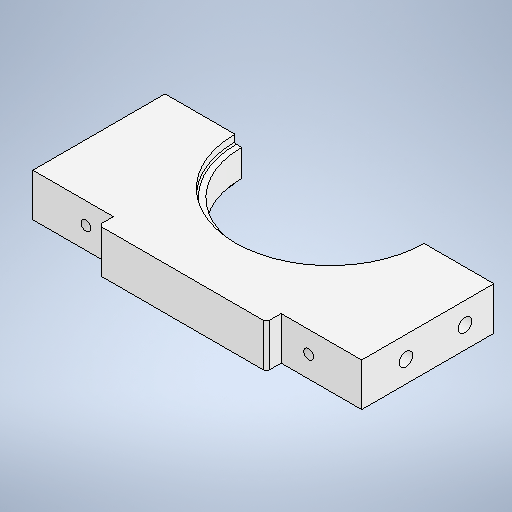
# Autodesk Inventor part: joint3_frame2
Saved by Autodesk Inventor 2025.3 (Build 293356030, 356C)
## iProperties
Created: 2025-11-25
Part Number: joint3_frame2
Material: PLA filament
Document SubType Name: Modeling
Designer: MSI
Density: 1.2 g/cm^3
Appearance: 일반
Mass: 86.6574 g
Surface Area: 168.952 cm^2
Volume: 72.2145 cm^3
Author: MSI
Autodesk Inventor part; units mm, degrees
ref_plane "YZ Plane" through (0, 0, 0) normal (1, 0, 0) x (0, 1, 0)
ref_plane "XZ Plane" through (0, 0, 0) normal (0, 1, 0) x (-1, 0, 0)
ref_plane "XY Plane" through (0, 0, 0) normal (0, 0, 1) x (1, 0, 0)
sketch "스케치1" plane through (0, 0, 0) normal (0, 1, 0) x (-1, 0, 0)
  line L0 (123, 55) -> (-123, 55)
  line L1 (-123, 55) -> (-123, -55)
  line L2 (-123, -55) -> (123, -55)
  line L3 (123, -55) -> (123, 55)
  line L4 (123, 55) -> (-123, -55) construction
  line L5 (-123, 55) -> (123, -55) construction
  point P0 (0, 0)
  dimension "d0" = 110
  dimension "d1" = 246
  constraints: 12 end point, 2 midpoint, 2 parallel, 1 horizontal, 1 perpendicular
  measures "d0" distance of L0.end L1.end
  measures "d1" distance of L0.start L0.end
extrude "돌출1" add sketch "스케치1" along normal mid plane 16
sketch "스케치2" plane through (0, 8, 0) normal (0, 1, 0) x (1, 0, 0)
  point P0 (0, 0)
hole "구멍1" at (0, 8, 0) direction (0, -1, 0) diameter 65.5 end through all counterbore diameter 70.5 counterbore depth 3
mirror "미러1" about plane through (0, 0, 0) normal (0, 1, 0) of "구멍1"
sketch "스케치3" plane through (0, 8, 0) normal (0, 1, 0) x (1, 0, 0)
  line L0 (-123, 55) -> (-123, -55) projected
  line L1 (-123, 40) -> (-112.5, 40)
  line L2 (-112.5, 40) -> (-112.5, -40)
  line L3 (-112.5, -40) -> (-123, -40)
  line L4 (-123, -40) -> (-123, 40)
  line L5 (-123, -55) -> (123, -55) projected
  point P0 (0, 0)
  point P1 (-123, 0)
  dimension "d12" = 10.5
  dimension "d13" = 15
  constraints: 8 end point, 2 midpoint, 2 parallel, 1 horizontal, 1 perpendicular, 1 point on line
  measures "d12" distance of L2.end L3.end
  measures "d13" distance between parallel lines of L5 L3
extrude "돌출2" cut sketch "스케치3" against normal through all
sketch "스케치4" plane through (-112.5, 8, -40) normal (-1, 0, 0) x (0, 0, 1)
  line L0 (10, -8) -> (70, -8) construction
  point P0 (40, -8)
  point P1 (40, -8)
  point P2 (50, -8)
  point P3 (30, -8)
  dimension "d21" = 20
  dimension "d22" = 60
  dimension "d23" = 20
  constraints: 3 coincident, 2 end point, 2 point on line, 1 horizontal, 1 midpoint
  measures "d21" distance of point (30, -8) point (10, -8)
  measures "d22" distance of L0.start L0.end
  measures "d23" distance of L0.end point (50, -8)
hole "구멍2" at (-112.5, 0, -30) at (-112.5, 0, 30) at (-112.5, 0, 10) at (-112.5, 0, -10) direction (1, 0, 0) diameter 3.6881 depth 8 tip angle 118 thread size "M4.5x0.75" class "6H" standard "ISO Metric profile"
sketch "스케치5" plane through (0, 8, 0) normal (0, 1, 0) x (1, 0, 0)
  line L0 (-118, 47.5) -> (-118, -47.5) construction
  line L1 (123, 55) -> (-123, 55) projected
  line L2 (-123, -40) -> (-123, -55) projected
  point P0 (0, 0)
  point P1 (-118, 0)
  dimension "d31" = 7.5
  dimension "d32" = 5
  constraints: 2 coincident, 2 end point, 1 horizontal alignment, 1 midpoint, 1 vertical
  measures "d31" distance from line of L0.start L1
  measures "d32" distance between parallel lines of L0 L2
hole "구멍3" at (-118, 8, -47.5) at (-118, 8, 47.5) direction (0, -1, 0) diameter 4.5 end through all counterbore diameter 8 counterbore depth 4.6 clearance for "Socket Head Cap Screw ISO 4762" size "M4" standard "ISO"
mirror "미러2" about plane through (0, 0, 0) normal (1, 0, 0) of "돌출2", "구멍2", "구멍3"
chamfer "모따기1" distance 1 angle 45 4 edges at (123, 0, -40) (123, 0, 40) (-123, 0, -40) (-123, 0, 40)
fillet "모깎기1" radius 0.5 2 edges at (0, 5, -35.25) (0, -5, -35.25)
fillet "모깎기2" radius 3 4 edges at (-123, 0, 55) (123, 0, 55) (123, 0, -55) (-123, 0, -55)
sketch "스케치6" plane through (-120, 8, 55) normal (0, 0, 1) x (1, 0, 0)
  line L0 (0, 0) -> (240, 0) projected
  line L1 (240, -16) -> (0, -16) projected
  line L2 (28.25, 0) -> (88.75, 0)
  line L3 (88.75, 0) -> (88.75, -16)
  line L4 (88.75, -16) -> (28.25, -16)
  line L5 (28.25, -16) -> (28.25, 0)
  point P0 (120, -8)
  point P1 (58.5, 0)
  point P2 (28.25, -16)
  dimension "d40" = 61.5
  dimension "d41" = 60.5
  constraints: 8 end point, 2 parallel, 2 point on line, 1 horizontal, 1 midpoint, 1 perpendicular
  measures "d40" horizontal distance of point (120, -8) point (58.5, 0)
  measures "d41" distance between parallel lines of L3 L5
extrude "돌출3" cut sketch "스케치6" against normal blind 5.5
sketch "스케치7" plane through (-120, 8, 49.5) normal (0, 0, 1) x (1, 0, 0)
  line L0 (38.5, -8) -> (78.5, -8) construction
  line L1 (28.25, 0) -> (88.75, 0) projected
  line L2 (28.25, -16) -> (28.25, 0) projected
  point P0 (120, -8)
  point P1 (58.5, -8)
  point P2 (58.5, 0)
  point P3 (28.25, -8)
  dimension "d47" = 40
  constraints: 3 midpoint, 2 coincident, 2 end point, 1 horizontal, 1 point on line, 1 vertical alignment
  measures "d47" distance of L0.start L0.end
hole "구멍4" at (-81.5, 0, 49.5) at (-41.5, 0, 49.5) direction (0, 0, -1) diameter 3.6881 depth 13 tip angle 118 thread size "M4.5x0.75" class "6H" standard "ISO Metric profile"
mirror "미러3" about plane through (0, 0, 0) normal (0, 0, 1) of "구멍4", "돌출3"
mirror "미러4" about plane through (0, 0, 0) normal (1, 0, 0) of "구멍4", "돌출3", "미러3"
chamfer "모따기3" distance 1 angle 45 8 edges at (-91.75, 0, 55) (-31.25, 0, 55) (31.25, 0, 55) (91.75, 0, 55) (-91.75, 0, -55) (-31.25, 0, -55) (31.25, 0, -55) (91.75, 0, -55)
sketch "스케치8" plane through (0, 8, 0) normal (0, 1, 0) x (1, 0, 0)
  line L0 (-61.25, -0.25) -> (61.25, -0.25)
  line L1 (61.25, -0.25) -> (61.25, -81.9376)
  line L2 (61.25, -81.9376) -> (-61.25, -81.9376)
  line L3 (-61.25, -81.9376) -> (-61.25, -0.25)
  line L4 (-91.75, -49.5) -> (-31.25, -49.5) projected
  line L5 (-61.5, -49.5) -> (-61.5, 49.5) construction
  line L6 (-91.75, 49.5) -> (-31.25, 49.5) projected
  line L7 (31.25, -49.5) -> (91.75, -49.5) projected
  line L8 (61.5, -49.5) -> (61.5, 49.5)
  line L9 (91.75, 49.5) -> (31.25, 49.5) projected
  point P0 (0, 0)
  dimension "d71" = 0.5
  dimension "d72" = 0.5
  dimension "d73" = 0.25
  constraints: 12 end point, 4 midpoint, 2 parallel, 1 horizontal, 1 perpendicular
  measures "d71" diameter of L3 L5
  measures "d72" diameter of L1 L8
  measures "d73" distance from line of point (0, 0) L0
extrude "돌출4" cut sketch "스케치8" against normal through all keep common part
sketch "스케치9" plane through (-61.25, 8, 49.5) normal (-1, 0, 0) x (0, 0, 1)
  line L0 (-82.5, -8) -> (-16.5, -8) construction
  point P0 (-49.5, -8)
  point P1 (-49.5, -8)
  point P2 (-60.5, -8)
  point P3 (-38.5, -8)
  dimension "d61" = 22
  dimension "d62" = 66
  dimension "d63" = 22
  constraints: 3 coincident, 2 end point, 2 point on line, 1 horizontal, 1 midpoint
  measures "d61" distance of point (-60.5, -8) L0.start
  measures "d62" distance of L0.start L0.end
  measures "d63" distance of L0.end point (-38.5, -8)
hole "구멍5" at (-61.25, 0, -33) at (-61.25, 0, -11) at (-61.25, 0, 11) at (-61.25, 0, 33) direction (1, 0, 0) diameter 5 depth 10 tip angle 118
mirror "미러5" about plane through (0, 0, 0) normal (1, 0, 0) of "구멍5"
sketch "스케치10" plane through (61.25, 8, 0.25) normal (0, 0, -1) x (-1, 0, 0)
  line L0 (20, -8) -> (102.5, -8) construction
  line L1 (0, 0) -> (0, -16) projected
  point P0 (61.25, -8)
  point P1 (61.25, -8)
  dimension "d74" = 20
  constraints: 3 coincident, 2 end point, 1 horizontal, 1 midpoint
  measures "d74" distance from line of L0.start L1
hole "구멍6" at (41.25, 0, 0.25) at (-41.25, 0, 0.25) direction (0, 0, 1) diameter 5 depth 10 tip angle 118
equation "\"d22\" = 3 * d21"
equation "\"d23\" = d21"
equation "\"d72\" = d71"
equation "\"d62\" = 3 * d61"
equation "\"d63\" = d61"
